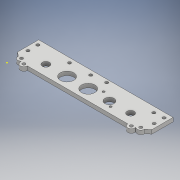
# Autodesk Inventor part: 1枚目
Saved by Autodesk Inventor 2018 (Build 220112000, 112)
## iProperties
Created: 2018-08-16
Part Number: 1枚目
Material: 一般
Document SubType Name: Modeling
Designer: shun2
Density: 1 g/cm^3
Appearance: 既定
Author: shun2
Autodesk Inventor part; units mm, degrees
ref_plane "YZ Plane" through (0, 0, 0) normal (1, 0, 0) x (0, 1, 0)
ref_plane "XZ Plane" through (0, 0, 0) normal (0, 1, 0) x (-1, 0, 0)
ref_plane "XY Plane" through (0, 0, 0) normal (0, 0, 1) x (1, 0, 0)
sketch "スケッチ1" plane through (0, 0, 0) normal (0, 0, 1) x (1, 0, 0)
  circle A0 centre (10.6603, 9.9994) radius 2.15
  circle A1 centre (179.6946, 9.9994) radius 2.15
  circle A2 centre (100.6774, 40.6494) radius 2.15
  circle A3 centre (80.1774, 38.4994) radius 2.15
  circle A4 centre (50.1774, 38.4994) radius 2.15
  circle A5 centre (19.0782, 4.9994) radius 2.15
  circle A6 centre (171.2766, 4.9994) radius 2.15
  circle A7 centre (171.0615, 37.0055) radius 2.15
  circle A8 centre (5.8155, 23.9994) radius 2.15
  circle A9 centre (5.8155, 37.9994) radius 2.15
  circle A10 centre (184.5394, 23.9994) radius 2.15
  circle A11 centre (184.5394, 37.9994) radius 2.15
  circle A12 centre (155.1774, 19.9994) radius 5
  circle A13 centre (95.1774, 19.9994) radius 9.5
  circle A14 centre (65.1774, 19.9994) radius 9.5
  circle A15 centre (35.1774, 19.9994) radius 5
  circle A16 centre (132.9274, 13.826) radius 1.6
  circle A17 centre (109.6774, 27.2494) radius 1.6
  line L0 (105.6774, 48.2494) -> (144.6774, 48.2494)
  line L1 (144.6774, 48.2494) -> (144.6774, 27.2494)
  arc A18 (105.6774, 27.2494) -> (144.6774, 27.2494) centre (125.1774, 27.2494) ccw
  line L2 (105.6774, 27.2494) -> (105.6774, 48.2494)
  circle A19 centre (125.1774, 19.9994) radius 6.5
  line L3 (0, 44.9994) -> (0, 14.9994)
  line L4 (0, 14.9994) -> (5.6908, 10.5508)
  arc A20 (5.6908, 10.5508) -> (13.7466, 6.0657) centre (10.6603, 9.9994) ccw
  line L5 (13.7466, 6.0657) -> (14.154, 5.8665)
  arc A21 (14.154, 5.8665) -> (24.0782, 4.9994) centre (19.0782, 4.9994) ccw
  line L6 (190.3548, 44.9994) -> (190.3548, 14.9994)
  line L7 (190.3548, 14.9994) -> (184.6641, 10.5508)
  arc A22 (176.6082, 6.0657) -> (184.6641, 10.5508) centre (179.6946, 9.9994) ccw
  line L8 (176.6082, 6.0657) -> (176.2009, 5.8665)
  arc A23 (166.2766, 4.9994) -> (176.2009, 5.8665) centre (171.2766, 4.9994) ccw
  line L9 (24.0782, 4.9994) -> (166.2766, 4.9994)
  line L10 (0, 44.9994) -> (190.3548, 44.9994)
  line L11 (0, 44.9994) -> (190.3548, 44.9994)
  line L12 (190.3548, 44.9994) -> (190.3548, 14.9994)
  line L13 (0, 44.9994) -> (0, 14.9994)
  line L14 (5.6908, 10.5508) -> (0, 14.9994)
  line L15 (24.0782, 4.9994) -> (166.2766, 4.9994)
  line L16 (184.6641, 10.5508) -> (190.3548, 14.9994)
  arc A24 (8.228, 5.6308) -> (13.7466, 6.0657) centre (10.6603, 9.9994) ccw
  line L17 (13.7466, 6.0657) -> (14.154, 5.8665)
  arc A25 (166.2766, 4.9994) -> (176.2009, 5.8665) centre (171.2766, 4.9994) ccw
  arc A26 (176.6082, 6.0657) -> (184.6641, 10.5508) centre (179.6946, 9.9994) ccw
  line L18 (176.6082, 6.0657) -> (176.2009, 5.8665)
  arc A27 (16.5868, 0.6644) -> (24.0782, 4.9994) centre (19.0782, 4.9994) ccw
  circle A28 centre (5.8155, 37.9994) radius 2.15
  circle A29 centre (5.8155, 23.9994) radius 2.15
  circle A30 centre (10.6603, 9.9994) radius 2.15
  circle A31 centre (19.0782, 4.9994) radius 2.15
  circle A32 centre (50.1774, 38.4994) radius 2.15
  circle A33 centre (80.1774, 38.4994) radius 2.15
  circle A34 centre (100.6774, 40.6494) radius 2.15
  circle A35 centre (171.0615, 37.0055) radius 2.15
  circle A36 centre (184.5394, 37.9994) radius 2.15
  circle A37 centre (184.5394, 23.9994) radius 2.15
  circle A38 centre (179.6946, 9.9994) radius 2.15
  circle A39 centre (171.2766, 4.9994) radius 2.15
  circle A40 centre (109.6774, 27.2494) radius 1.6
  circle A41 centre (132.9274, 13.826) radius 1.6
  circle A42 centre (125.1774, 19.9994) radius 6.5
  point P0 (0, 0)
  dimension "d0" = 10
  dimension "d1" = 19
  constraints: 43 centre point, 38 end point, 20 point on circle, 15 coincident, 15 concentric, 6 collinear, 1 perpendicular
  measures "d0" diameter of A15
  measures "d1" diameter of A14
sketch "スケッチ2" plane through (0, 0, 0) normal (0, 0, 1) x (1, 0, 0)
  point P0 (0, 0)
extrude "押し出し1" add sketch "スケッチ1" along normal blind 5.5 contours L10 L1 A18 L2 | L2 A18 L1 L10 L6 L7 A22 L8 A23 L9 A21 L5 A20 L4 L3
